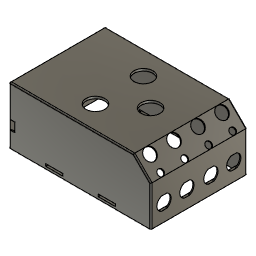
Main_case (Autodesk Fusion 360 design; units mm, degrees)
Autodesk Fusion 360 part; units mm, degrees
note: some values were not read from the file. Set by a fixed rule: which sketch regions a step uses.
sketch "Sketch1" plane through (0, 0, 0) normal (0, 0, 1) x (1, 0, 0)
  line L0 (0, 0) -> (120, 0)
  line L1 (120, 0) -> (120, 80)
  line L2 (120, 80) -> (0, 80)
  line L3 (0, 80) -> (0, 0)
  line L4 (-2, -2) -> (-2, 82)
  line L5 (-2, 82) -> (122, 82)
  line L6 (122, 82) -> (122, -2)
  line L7 (122, -2) -> (-2, -2)
  constraint horizontal L0
  constraint vertical L1
  constraint horizontal L2
  constraint vertical L3
  constraint coincident L0.start L3.end
  constraint perpendicular L4 L5
  constraint perpendicular L4 L7
extrude "Extrude1" add sketch "Sketch1" along normal blind 40 makes body 1
extrude "Extrude2" add 1 faces at (40, 81.3333, 40) along direction (0, 0, 1) blind 10 on bodies 1 bodies 1
sketch "Sketch2" plane through (0, -2, 0) normal (0, -1, 0) x (1, 0, 0)
  line L0 (-2, 0) -> (122, 0)
  line L1 (122, 0) -> (122, 50)
  line L2 (122, 50) -> (-2, 50)
  line L3 (-2, 50) -> (-2, 0)
  line L4 (122, 35) -> (107, 50)
  constraint coincident L2 L4.end
  constraint coincident L1 L4.start
extrude "Extrude3" cut sketch "Sketch2" against normal blind 135 contours L1 L2 L4 bodies 1
sketch "Sketch3" plane through (78.5, 0, 78.5) normal (0.707107, 0, 0.707107) x (0, 1, 0)
  line L0 (80, -40.3051) -> (80, -58.6899)
  line L1 (80, -58.6899) -> (0, -58.6899)
  line L2 (0, -58.6899) -> (0, -40.3051)
  line L3 (0, -40.3051) -> (-2, -40.3051)
  line L4 (-2, -40.3051) -> (-2, -61.5183)
  line L5 (-2, -61.5183) -> (82, -61.5183)
  line L6 (82, -61.5183) -> (82, -40.3051)
  line L7 (82, -40.3051) -> (80, -40.3051)
  line L8 (-2, -40.3051) -> (82, -40.3051)
  line L9 (82, -40.3051) -> (82, -61.5183)
  line L10 (82, -61.5183) -> (-2, -61.5183)
  line L11 (-2, -61.5183) -> (-2, -40.3051)
  constraint horizontal L8
  constraint vertical L9
  constraint horizontal L10
  constraint vertical L11
  constraint coincident L5.end L6.start
  constraint coincident L3.end L4.start
extrude "Extrude4" add sketch "Sketch3" against normal blind 2 bodies 1
sketch "Sketch4" plane through (0, 0, 50) normal (0, 0, 1) x (-1, 0, 0)
  line L0 (-107, -80) -> (-107, -82)
  line L1 (-107, -82) -> (2, -82)
  line L2 (2, -82) -> (2, 2)
  line L3 (2, 2) -> (-107, 2)
  line L4 (-107, 2) -> (-107, 0)
  line L5 (-107, 0) -> (0, 0)
  line L6 (0, 0) -> (0, -80)
  line L7 (0, -80) -> (-107, -80)
  line L8 (2, -82) -> (-107, -82)
  line L9 (-107, -82) -> (-107, 2)
  line L10 (-107, 2) -> (2, 2)
  line L11 (2, 2) -> (2, -82)
  constraint horizontal L8
  constraint vertical L9
  constraint horizontal L10
  constraint vertical L11
  constraint coincident L3.end L4.start
  constraint coincident L1.end L2.start
extrude "Extrude5" add sketch "Sketch4" against normal blind 2 bodies 1
sketch "Sketch5" plane through (78.5, 0, 78.5) normal (0.707107, 0, 0.707107) x (0, 1, 0)
  line L0 (82, -40.3051) -> (-2, -40.3051)
  line L1 (-2, -40.3051) -> (-2, -61.5183)
  line L2 (-2, -61.5183) -> (82, -61.5183)
  line L3 (82, -61.5183) -> (82, -40.3051)
  line L4 (-2, -40.3051) -> (-2, -61.5183)
  line L5 (-2, -40.3051) -> (-2, -50.9117)
  line L6 (40, -40.3051) -> (-2, -40.3051)
  line L7 (82, -40.3051) -> (40, -40.3051)
  line L8 (-2, -40.3051) -> (19, -40.3051)
  circle A0 centre (8.5, -58.7683) radius 2.75
  circle A1 centre (8.5, -45.5551) radius 5.25
  line L9 (19, -40.3051) -> (40, -40.3051)
  circle A2 centre (29.5, -45.5551) radius 5.25
  circle A3 centre (29.5, -58.7683) radius 2.75
  line L10 (40, -40.3051) -> (61, -40.3051)
  line L11 (61, -40.3051) -> (82, -40.3051)
  circle A4 centre (50.5, -45.5551) radius 5.25
  circle A5 centre (50.5, -58.7683) radius 2.75
  circle A6 centre (71.5, -45.5551) radius 5.25
  circle A7 centre (71.5, -58.7683) radius 2.75
  dimension "d13" = 5.5
  dimension "d14" = 10.5
  dimension "d15" = 10.5
  dimension "d16" = 5.5
  dimension "d17" = 10.5
  dimension "d18" = 5.5
  dimension "d19" = 10.5
  dimension "d20" = 5.5
  constraint coincident L0.end L1.start
  constraint coincident L1.end L2.start
  constraint midpoint L4 L5.end
  constraint midpoint L0 L6.start
  constraint midpoint L6 L8.end
  constraint coincident L0.start L3.end
  constraint midpoint L7 L10.end
  measures "d13" diameter of A0
  measures "d14" diameter of A1
  measures "d15" diameter of A2
  measures "d16" diameter of A3
  measures "d17" diameter of A4
  measures "d18" diameter of A5
  measures "d19" diameter of A6
  measures "d20" diameter of A7
extrude "Extrude6" cut sketch "Sketch5" against normal blind 20 contours A6 | A4 | A2 | A1 | A0 | A3 | A5 | A7 bodies 1
chamfer "Chamfer1" distance 1 angle 45 16 edges at (105, 71.5, 48) (113.0104, 71.5, 41.1612) (116.6967, 71.5, 37.4749) (120, 71.5, 33) (105, 50.5, 48) (113.0104, 50.5, 41.1612) (116.6967, 50.5, 37.4749) (120, 50.5, 33) (105, 29.5, 48) (113.0104, 29.5, 41.1612) (116.6967, 29.5, 37.4749) (120, 29.5, 33) (105, 8.5, 48) (113.0104, 8.5, 41.1612) (116.6967, 8.5, 37.4749) (120, 8.5, 33) on bodies 1
sketch "Sketch6" plane through (120, 0, 0) normal (-1, 0, 0) x (0, -1, 0)
  spline S0 degree 3 poles (-11.6272, 34.1716) (-11.364, 33.6522) (-11.0186, 33.1887) (-10.2377, 32.5093) (-9.8211, 32.2678) (-9.0887, 32.0448) (-8.7945, 32) (-8.5, 32) (-8.2055, 32) (-7.9113, 32.0448) (-7.1789, 32.2678) (-6.7623, 32.5093) (-5.9814, 33.1887) (-5.636, 33.6522) (-5.3728, 34.1716) knots -0.948969 -0.948969 -0.948969 -0.948969 -0.551543 -0.551543 -0.212132 -0.212132 0 0 0 0.212132 0.212132 0.551543 0.551543 0.948969 0.948969 0.948969 0.948969
  spline S1 degree 3 poles (-11.6784, 34.2753) (-11.6617, 34.2405) (-11.6446, 34.2059) (-11.6272, 34.1716) knots -0.975231 -0.975231 -0.975231 -0.975231 -0.948969 -0.948969 -0.948969 -0.948969
  spline S2 degree 2 poles (-11.7203, 34.1716) (-11.6993, 34.2238) (-11.6784, 34.2753) knots -18.7019 -18.7019 -18.7019 -18.668651 -18.668651 -18.668651 weights 1.000003 1.000003 1.000003
  line L0 (-11.7203, 34.1716) -> (-26.2797, 34.1716)
  spline S3 degree 2 poles (-26.3216, 34.2753) (-26.3007, 34.2238) (-26.2797, 34.1716) knots -13.625289 -13.625289 -13.625289 -13.59204 -13.59204 -13.59204 weights 1.000003 1.000003 1.000003
  spline S4 degree 3 poles (-26.3216, 34.2753) (-26.3383, 34.2405) (-26.3554, 34.2059) (-26.3728, 34.1716) knots -0.975231 -0.975231 -0.975231 -0.975231 -0.948969 -0.948969 -0.948969 -0.948969
  spline S5 degree 3 poles (-32.6272, 34.1716) (-32.364, 33.6522) (-32.0186, 33.1887) (-31.2377, 32.5093) (-30.8211, 32.2678) (-30.0887, 32.0448) (-29.7945, 32) (-29.5, 32) (-29.2055, 32) (-28.9113, 32.0448) (-28.1789, 32.2678) (-27.7623, 32.5093) (-26.9814, 33.1887) (-26.636, 33.6522) (-26.3728, 34.1716) knots -0.948969 -0.948969 -0.948969 -0.948969 -0.551543 -0.551543 -0.212132 -0.212132 0 0 0 0.212132 0.212132 0.551543 0.551543 0.948969 0.948969 0.948969 0.948969
  spline S6 degree 3 poles (-32.6784, 34.2753) (-32.6617, 34.2405) (-32.6446, 34.2059) (-32.6272, 34.1716) knots -0.975231 -0.975231 -0.975231 -0.975231 -0.948969 -0.948969 -0.948969 -0.948969
  spline S7 degree 2 poles (-32.7203, 34.1716) (-32.6993, 34.2238) (-32.6784, 34.2753) knots -18.7019 -18.7019 -18.7019 -18.668651 -18.668651 -18.668651 weights 1.000003 1.000003 1.000003
  line L1 (-32.7203, 34.1716) -> (-47.2797, 34.1716)
  spline S8 degree 2 poles (-47.3216, 34.2753) (-47.3007, 34.2238) (-47.2797, 34.1716) knots -13.625289 -13.625289 -13.625289 -13.59204 -13.59204 -13.59204 weights 1.000003 1.000003 1.000003
  spline S9 degree 3 poles (-47.3216, 34.2753) (-47.3383, 34.2405) (-47.3554, 34.2059) (-47.3728, 34.1716) knots -0.975231 -0.975231 -0.975231 -0.975231 -0.948969 -0.948969 -0.948969 -0.948969
  spline S10 degree 3 poles (-53.6272, 34.1716) (-53.364, 33.6522) (-53.0186, 33.1887) (-52.2377, 32.5093) (-51.8211, 32.2678) (-51.0887, 32.0448) (-50.7945, 32) (-50.5, 32) (-50.2055, 32) (-49.9113, 32.0448) (-49.1789, 32.2678) (-48.7623, 32.5093) (-47.9814, 33.1887) (-47.636, 33.6522) (-47.3728, 34.1716) knots -0.948969 -0.948969 -0.948969 -0.948969 -0.551543 -0.551543 -0.212132 -0.212132 0 0 0 0.212132 0.212132 0.551543 0.551543 0.948969 0.948969 0.948969 0.948969
  spline S11 degree 3 poles (-53.6784, 34.2753) (-53.6617, 34.2405) (-53.6446, 34.2059) (-53.6272, 34.1716) knots -0.975231 -0.975231 -0.975231 -0.975231 -0.948969 -0.948969 -0.948969 -0.948969
  spline S12 degree 2 poles (-53.7203, 34.1716) (-53.6993, 34.2238) (-53.6784, 34.2753) knots -18.7019 -18.7019 -18.7019 -18.668651 -18.668651 -18.668651 weights 1.000003 1.000003 1.000003
  line L2 (-53.7203, 34.1716) -> (-68.2797, 34.1716)
  spline S13 degree 2 poles (-68.3216, 34.2753) (-68.3007, 34.2238) (-68.2797, 34.1716) knots -13.625289 -13.625289 -13.625289 -13.59204 -13.59204 -13.59204 weights 1.000003 1.000003 1.000003
  spline S14 degree 3 poles (-68.3216, 34.2753) (-68.3383, 34.2405) (-68.3554, 34.2059) (-68.3728, 34.1716) knots -0.975231 -0.975231 -0.975231 -0.975231 -0.948969 -0.948969 -0.948969 -0.948969
  spline S15 degree 3 poles (-74.6272, 34.1716) (-74.364, 33.6522) (-74.0186, 33.1887) (-73.2377, 32.5093) (-72.8211, 32.2678) (-72.0887, 32.0448) (-71.7945, 32) (-71.5, 32) (-71.2055, 32) (-70.9113, 32.0448) (-70.1789, 32.2678) (-69.7623, 32.5093) (-68.9814, 33.1887) (-68.636, 33.6522) (-68.3728, 34.1716) knots -0.948969 -0.948969 -0.948969 -0.948969 -0.551543 -0.551543 -0.212132 -0.212132 0 0 0 0.212132 0.212132 0.551543 0.551543 0.948969 0.948969 0.948969 0.948969
  spline S16 degree 3 poles (-74.6784, 34.2753) (-74.6617, 34.2405) (-74.6446, 34.2059) (-74.6272, 34.1716) knots -0.975231 -0.975231 -0.975231 -0.975231 -0.948969 -0.948969 -0.948969 -0.948969
  spline S17 degree 2 poles (-74.7203, 34.1716) (-74.6993, 34.2238) (-74.6784, 34.2753) knots -18.7019 -18.7019 -18.7019 -18.668651 -18.668651 -18.668651 weights 1.000003 1.000003 1.000003
  line L3 (-74.7203, 34.1716) -> (-80, 34.1716)
  line L4 (-80, 34.1716) -> (-80, 0)
  line L5 (-80, 0) -> (0, 0)
  line L6 (0, 0) -> (0, 34.1716)
  line L7 (0, 34.1716) -> (-5.2797, 34.1716)
  spline S18 degree 2 poles (-5.3216, 34.2753) (-5.3007, 34.2238) (-5.2797, 34.1716) knots -13.625289 -13.625289 -13.625289 -13.59204 -13.59204 -13.59204 weights 1.000003 1.000003 1.000003
  spline S19 degree 3 poles (-5.3216, 34.2753) (-5.3383, 34.2405) (-5.3554, 34.2059) (-5.3728, 34.1716) knots -0.975231 -0.975231 -0.975231 -0.975231 -0.948969 -0.948969 -0.948969 -0.948969
  circle A0 centre (-70.5, 15) radius 6.25
  circle A1 centre (-50.5, 15) radius 6.25
  circle A2 centre (-29.5, 15) radius 6.25
  circle A3 centre (-9.5, 15) radius 6.25
  line L8 (-63.25, 9.25) -> (-77.75, 9.25)
  line L9 (-77.75, 9.25) -> (-77.75, 20.75)
  line L10 (-77.75, 20.75) -> (-63.25, 20.75)
  line L11 (-63.25, 20.75) -> (-63.25, 9.25)
  line L12 (-43.25, 9.25) -> (-57.75, 9.25)
  line L13 (-57.75, 9.25) -> (-57.75, 20.75)
  line L14 (-57.75, 20.75) -> (-43.25, 20.75)
  line L15 (-43.25, 20.75) -> (-43.25, 9.25)
  line L16 (-22.25, 9.25) -> (-36.75, 9.25)
  line L17 (-36.75, 9.25) -> (-36.75, 20.75)
  line L18 (-36.75, 20.75) -> (-22.25, 20.75)
  line L19 (-22.25, 20.75) -> (-22.25, 9.25)
  line L20 (-2.25, 9.25) -> (-16.75, 9.25)
  line L21 (-16.75, 9.25) -> (-16.75, 20.75)
  line L22 (-16.75, 20.75) -> (-2.25, 20.75)
  line L23 (-2.25, 20.75) -> (-2.25, 9.25)
  point P0 (-70.5, 15)
  point P1 (-50.5, 15)
  point P2 (-29.5, 15)
  point P3 (-9.5, 15)
  constraint horizontal L8
  constraint perpendicular L8 L9
  constraint parallel L8 L10
  constraint parallel L9 L11
  constraint horizontal L12
  constraint perpendicular L12 L13
  constraint parallel L12 L14
  constraint parallel L13 L15
  constraint coincident P1 A1.centre
  constraint horizontal L16
  constraint perpendicular L16 L17
  constraint parallel L16 L18
  constraint parallel L17 L19
  constraint coincident P2 A2.centre
  constraint horizontal L20
  constraint perpendicular L20 L21
  constraint parallel L20 L22
  constraint parallel L21 L23
  constraint coincident P3 A3.centre
extrude "Extrude7" cut sketch "Sketch6" against normal blind 51 contours A0 L8 L10 | A1 L12 L14 | A2 L16 L18 | A3 L20 L22 bodies 1
extrude "Extrude8" cut sketch "Sketch6" against normal blind 1 contours A0 L8 L10 L11 | A0 L8 L9 L10 | A1 L12 L14 L15 | A1 L12 L13 L14 | A2 L16 L18 L19 | A2 L16 L17 L18 | A3 L20 L22 L23 | A3 L20 L21 L22 bodies 1
sketch "Sketch7" plane through (0, 0, 50) normal (0, 0, 1) x (-1, 0, 0)
  line L0 (-107, 2) -> (-107, -8.5)
  line L1 (-107, -8.5) -> (-107, -29.5)
  line L2 (-107, -29.5) -> (-107, -50.5)
  line L3 (-107, -50.5) -> (-107, -71.5)
  line L4 (-107, -71.5) -> (-107, -82)
  line L5 (-107, -82) -> (2, -82)
  line L6 (2, -82) -> (2, 2)
  line L7 (2, 2) -> (-107, 2)
  line L8 (-107, -82) -> (-107, 2)
  line L9 (-107, -40) -> (2, -40)
  line L10 (-52.5, -40) -> (-52.5, 2)
  line L11 (-52.5, -40) -> (-52.5, -82)
  circle A0 centre (-52.5, -61) radius 8.25
  circle A1 centre (-52.5, -19) radius 8.25
  line L12 (-107, -40) -> (-52.5, -40)
  circle A2 centre (-79.75, -40) radius 8.25
  dimension "d42" = 16.5
  dimension "d43" = 16.5
  dimension "d75" = 16.5
  constraint coincident L4.end L5.start
  constraint coincident L0.start L7.end
  constraint midpoint L8 L9.start
  constraint midpoint L6 L9.end
  constraint midpoint L9 L10.start
  constraint midpoint L7 L10.end
  constraint midpoint L5 L11.end
  constraint midpoint L11 A0.centre
  constraint midpoint L10 A1.centre
  constraint midpoint L12 A2.centre
  measures "d42" diameter of A0
  measures "d43" diameter of A1
  measures "d75" diameter of A2
extrude "Extrude9" cut sketch "Sketch7" against normal blind 30 contours L10 A1 | L10 A1 | L11 A0 | L11 A0 bodies 1
sketch "Sketch8" plane through (0, 0, 0) normal (1, 0, 0) x (0, 1, 0)
  line L0 (80, 48) -> (0, 48)
  line L1 (0, 48) -> (0, 0)
  line L2 (0, 0) -> (80, 0)
  line L3 (80, 0) -> (80, 48)
  line L4 (10, 26.75) -> (0, 26.75)
  line L5 (10, 9.25) -> (0, 9.25)
  line L6 (0, 26.75) -> (27.5, 26.75)
  line L7 (0, 9.25) -> (27.5, 9.25)
  line L8 (27.5, 26.75) -> (27.5, 9.25)
  line L9 (27.5, 26.75) -> (22.4893, 26.75)
  line L10 (22.4893, 26.75) -> (22.4893, 9.25)
  line L11 (22.4893, 9.25) -> (27.5, 9.25)
  line L12 (27.5, 9.25) -> (27.5, 26.75)
  line L13 (27.5, 18) -> (0, 18)
  line L14 (27.5, 18) -> (80, 18)
  line L15 (80, 18) -> (80, 27.75)
  line L16 (80, 18) -> (80, 8.25)
  line L17 (80, 18) -> (80, 23.5)
  line L18 (80, 18) -> (80, 12.5)
  dimension "d48" = 27.5
  dimension "d49" = 27.5
  dimension "d60" = 9.75
  dimension "d61" = 9.75
  dimension "d62" = 5.5
  dimension "d63" = 5.5
  constraint coincident L1 L4.end
  constraint perpendicular L1 L4
  constraint coincident L1 L5.end
  constraint perpendicular L1 L5
  constraint perpendicular L1 L6
  constraint perpendicular L1 L7
  constraint horizontal L9
  constraint vertical L10
  constraint horizontal L11
  constraint vertical L12
  constraint coincident L7 L10.end
  constraint midpoint L12 L13.start
  constraint coincident L1 L13.end
  constraint perpendicular L1 L13
  constraint coincident L3 L14.end
  constraint perpendicular L3 L14
  constraint perpendicular L14 L15
  constraint perpendicular L14 L16
  constraint perpendicular L14 L17
  constraint perpendicular L14 L18
  measures "d48" distance of L4.end L6.end
  measures "d49" distance of L5.end L7.end
  measures "d60" distance of L14.end L15.end
  measures "d61" distance of L14.end L16.end
  measures "d62" distance of L14.end L17.end
  measures "d63" distance of L14.end L18.end
extrude "Extrude10" cut sketch "Sketch8" against normal blind 1.2 contours L7 L8 L10 L11 L12 L13 | L6 L8 L9 L10 L12 L13 bodies 1
extrude "Extrude11" cut sketch "Sketch8" against normal blind 1 contours L1 L4 L6 L10 L13 | L1 L5 L7 L10 L13 bodies 1
sketch "Sketch9" plane through (0, 0, 0) normal (0, 1, 0) x (-1, 0, 0)
  line L0 (0, 48) -> (-106.1716, 48)
  line L1 (-106.1716, 48) -> (-120, 34.1716)
  line L2 (-120, 34.1716) -> (-120, 0)
  line L3 (-120, 0) -> (0, 0)
  line L4 (0, 0) -> (0, 9.25)
  line L5 (0, 9.25) -> (1, 9.25)
  line L6 (1, 9.25) -> (1, 26.75)
  line L7 (1, 26.75) -> (0, 26.75)
  line L8 (0, 26.75) -> (0, 48)
  line L9 (1, 26.75) -> (-3, 26.75)
  line L10 (-3, 26.75) -> (-3, 9.25)
  line L11 (-3, 9.25) -> (1, 9.25)
  line L12 (1, 9.25) -> (1, 26.75)
  line L13 (1, 18) -> (1, 22)
  line L14 (1, 18) -> (1, 14)
  line L15 (1, 22) -> (-3, 22)
  line L16 (1, 14) -> (-3, 14)
  dimension "d54" = 4
  dimension "d55" = 17.5
  constraint horizontal L9
  constraint vertical L10
  constraint horizontal L11
  constraint vertical L12
  constraint coincident L6.end L7.start
  constraint midpoint L12 L13.start
  constraint coincident L6 L13.end
  constraint parallel L6 L13
  constraint coincident L12 L14.end
  constraint parallel L12 L14
  constraint coincident L10 L15.end
  constraint perpendicular L10 L15
  constraint coincident L10 L16.end
  constraint perpendicular L10 L16
  measures "d54" distance of L6.end L9.end
  measures "d55" distance of L6.end L5.end
extrude "Extrude12" cut sketch "Sketch9" against normal blind 1 contours L6 L7 L9 L10 L12 L15 | L5 L6 L10 L11 L12 L16 bodies 1
extrude "Extrude13" cut sketch "Sketch9" against normal blind 9 contours L6 L10 L12 L13 L14 L15 L16 bodies 1
sketch "Sketch10" plane through (0, 80, 0) normal (0, -1, 0) x (1, 0, 0)
  line L0 (106.1716, 48) -> (0, 48)
  line L1 (0, 48) -> (0, 0)
  line L2 (0, 0) -> (120, 0)
  line L3 (120, 0) -> (120, 34.1716)
  line L4 (120, 34.1716) -> (106.1716, 48)
  line L5 (0, 8.25) -> (3.5, 8.25)
  line L6 (0, 27.75) -> (3.5, 27.75)
  line L7 (0, 23.5) -> (3.5, 23.5)
  line L8 (0, 12.5) -> (3.5, 12.5)
  line L9 (3.5, 27.75) -> (3.5, 8.25)
  dimension "d67" = 3.5
  dimension "d68" = 3.5
  constraint coincident L1 L5.start
  constraint perpendicular L1 L5
  constraint coincident L1 L6.start
  constraint perpendicular L1 L6
  constraint coincident L1 L7.start
  constraint perpendicular L1 L7
  constraint coincident L1 L8.start
  constraint perpendicular L1 L8
  constraint perpendicular L5 L9
  measures "d67" distance of L7.start L7.end
  measures "d68" distance of L8.start L8.end
extrude "Extrude14" cut sketch "Sketch10" against normal blind 1 contours L1 L6 L7 L9 | L1 L5 L8 L9 bodies 1
extrude "Extrude15" cut sketch "Sketch10" against normal blind 10 contours L1 L7 L8 L9 bodies 1
sketch "Sketch11" plane through (0, 0, 0) normal (1, 0, 0) x (0, 1, 0)
  line L0 (27.5, 9.25) -> (0, 9.25)
  line L1 (0, 9.25) -> (0, 0)
  line L2 (0, 0) -> (80, 0)
  line L3 (80, 0) -> (80, 8.25)
  line L4 (80, 8.25) -> (81, 8.25)
  line L5 (81, 8.25) -> (81, 12.5)
  line L6 (81, 12.5) -> (82, 12.5)
  line L7 (82, 12.5) -> (82, 23.5)
  line L8 (82, 23.5) -> (81, 23.5)
  line L9 (81, 23.5) -> (81, 27.75)
  line L10 (81, 27.75) -> (80, 27.75)
  line L11 (80, 27.75) -> (80, 48)
  line L12 (80, 48) -> (0, 48)
  line L13 (0, 48) -> (0, 26.75)
  line L14 (0, 26.75) -> (27.5, 26.75)
  line L15 (27.5, 26.75) -> (27.5, 9.25)
  line L16 (81, 23.5) -> (76, 23.5)
  line L17 (76, 23.5) -> (76, 12.5)
  line L18 (76, 12.5) -> (81, 12.5)
  line L19 (81, 27.75) -> (80.5, 27.75)
  line L20 (80.5, 27.75) -> (80.5, 8.25)
  line L21 (81, 23.5) -> (81, 12.5)
  constraint coincident L8.end L9.start
  constraint perpendicular L9 L16
  constraint perpendicular L6 L17
  constraint coincident L5.end L6.start
  constraint perpendicular L5 L18
  constraint coincident L9.end L10.start
  constraint midpoint L10 L19.end
  constraint midpoint L4 L20.end
extrude "Extrude16" cut sketch "Sketch11" against normal blind 1 contours L4 L5 L18 L20 | L16 L18 L20 L21 | L16 L17 L18 L20 | L9 L10 L16 L19 L20 bodies 1
extrude "Extrude17" cut sketch "Sketch7" against normal blind 5 contours L9 L12 A2 | L9 L12 A2 bodies 1
extrude "Extrude18" add sketch "Sketch1" against normal blind 2 separate body contours L0 L1 L2 L3 | L4 L5 L6 L7 makes body 2
sketch "Sketch12" plane through (0, 0, 0) normal (0, 0, 1) x (1, 0, 0)
  line L0 (2, 78) -> (118, 78)
  line L1 (118, 78) -> (118, 2)
  line L2 (118, 2) -> (2, 2)
  line L3 (2, 2) -> (2, 78)
  line L4 (2, 78) -> (118, 78)
  line L5 (118, 78) -> (118, 2)
  line L6 (118, 2) -> (2, 2)
  line L7 (2, 2) -> (2, 78)
  constraint perpendicular L0 L1
  constraint perpendicular L1 L2
  constraint perpendicular L0 L3
  constraint horizontal L4
  constraint vertical L5
  constraint horizontal L6
  constraint vertical L7
extrude "Extrude19" add sketch "Sketch1" along normal blind 2 contours L0 L1 L2 L3 bodies 2
sketch "Sketch13" plane through (0, 0, 2) normal (0, 0, 1) x (-1, 0, 0)
  line L0 (0, -80) -> (0, 0)
  line L1 (0, 0) -> (-120, 0)
  line L2 (-120, 0) -> (-120, -80)
  line L3 (-120, -80) -> (0, -80)
  line L4 (-2, -78) -> (-118, -78)
  line L5 (-118, -78) -> (-118, -2)
  line L6 (-118, -2) -> (-2, -2)
  line L7 (-2, -2) -> (-2, -78)
  constraint horizontal L4
  constraint vertical L5
  constraint horizontal L6
  constraint vertical L7
extrude "Extrude20" cut sketch "Sketch13" against normal blind 2 contours L4 L5 L6 L7 bodies 2
fillet "Fillet1" radius 1 9 edges at (-2, 82, 25) (52.5, 82, 50) (-2, 40, 50) (52.5, -2, 50) (114.5, -2, 42.5) (114.5, 82, 42.5) (122, 82, 17.5) (122, -2, 17.5) (-2, -2, 25) on bodies 1
fillet "Fillet2" radius 1 8 edges at (-2, 82, -1) (-2, 40, -2) (60, 82, -2) (-2, -2, -1) (60, -2, -2) (122, -2, -1) (122, 40, -2) (122, 82, -1) on bodies 2
sketch "Sketch14" plane through (0, 0, 2) normal (0, 0, 1) x (-1, 0, 0)
  line L0 (-118, -78) -> (-118, -2)
  line L1 (-118, -2) -> (-2, -2)
  line L2 (-2, -2) -> (-2, -78)
  line L3 (-2, -78) -> (-118, -78)
  line L4 (0, -80) -> (0, 0)
  line L5 (0, 0) -> (-120, 0)
  line L6 (-120, 0) -> (-120, -80)
  line L7 (-120, -80) -> (0, -80)
  line L8 (-118, -40) -> (-118, -55)
  line L9 (-118, -40) -> (-118, -25)
  line L10 (-118, -25) -> (-120, -25)
  line L11 (-120, -25) -> (-120, -55)
  line L12 (-118, -55) -> (-120, -55)
  line L13 (-30, -2) -> (-45, -2)
  line L14 (-45, -2) -> (-45, 0)
  line L15 (-45, 0) -> (-30, 0)
  line L16 (-30, 0) -> (-30, -2)
  line L17 (-76, -2) -> (-91, -2)
  line L18 (-91, -2) -> (-91, 0)
  line L19 (-91, 0) -> (-76, 0)
  line L20 (-76, 0) -> (-76, -2)
  line L21 (-2, -40) -> (-2, -47.5)
  line L22 (-2, -47.5) -> (0, -47.5)
  line L23 (0, -47.5) -> (0, -32.5)
  line L24 (-2, -32.5) -> (0, -32.5)
  line L25 (-2, -32.5) -> (-2, -40)
  line L26 (-30, -80) -> (-45, -80)
  line L27 (-45, -80) -> (-45, -78)
  line L28 (-45, -78) -> (-30, -78)
  line L29 (-30, -78) -> (-30, -80)
  line L30 (-76, -80) -> (-91, -80)
  line L31 (-91, -80) -> (-91, -78)
  line L32 (-91, -78) -> (-76, -78)
  line L33 (-76, -78) -> (-76, -80)
  constraint midpoint L0 L8.start
  constraint coincident L0 L8.end
  constraint parallel L0 L8
  constraint coincident L0 L9.end
  constraint parallel L0 L9
  constraint coincident L6 L10.end
  constraint perpendicular L6 L10
  constraint coincident L6 L11.end
  constraint perpendicular L10 L11
  constraint perpendicular L11 L12
  constraint horizontal L13
  constraint vertical L14
  constraint horizontal L15
  constraint vertical L16
  constraint coincident L5 L14.end
  constraint coincident L1 L13.start
  constraint horizontal L17
  constraint vertical L18
  constraint horizontal L19
  constraint vertical L20
  constraint coincident L5 L18.end
  constraint coincident L1 L17.start
  constraint midpoint L2 L21.start
  constraint coincident L2 L21.end
  constraint parallel L2 L21
  constraint coincident L4 L22.end
  constraint perpendicular L4 L22
  constraint coincident L4 L23.end
  constraint perpendicular L22 L23
  constraint coincident L2 L24.start
  constraint perpendicular L23 L24
  constraint coincident L7 L26.start
  constraint coincident L7 L30.start
  constraint horizontal L26
  constraint vertical L27
  constraint horizontal L28
  constraint vertical L29
  constraint coincident L3 L27.end
  constraint horizontal L30
  constraint vertical L31
  constraint horizontal L32
  constraint vertical L33
  constraint coincident L3 L31.end
extrude "Extrude21" add sketch "Sketch14" along normal blind 2 contours L0 L6 L8 L9 L10 L11 L12 | L3 L7 L30 L31 L32 L33 | L3 L7 L26 L27 L28 L29 | L1 L5 L17 L18 L19 L20 | L2 L4 L21 L22 L23 L24 L25 | L1 L5 L13 L14 L15 L16 bodies 2
sketch "Sketch15" plane through (120, 0, 0) normal (1, 0, 0) x (0, 1, 0)
  line L0 (0, 0) -> (80, 0)
  line L1 (80, 0) -> (80, 2)
  line L2 (80, 2) -> (55, 2)
  line L3 (55, 2) -> (55, 4)
  line L4 (55, 4) -> (25, 4)
  line L5 (25, 4) -> (25, 2)
  line L6 (25, 2) -> (0, 2)
  line L7 (0, 2) -> (0, 0)
  line L8 (25, 2) -> (55, 2)
  constraint coincident L5.end L6.start
  constraint coincident L2.end L3.start
extrude "Extrude22" add sketch "Sketch15" along normal blind 1 contours L3 L4 L5 L8 bodies 2
sketch "Sketch16" plane through (0, 0, 0) normal (0, -1, 0) x (1, 0, 0)
  line L0 (0, 0) -> (120, 0)
  line L1 (120, 0) -> (120, 2)
  line L2 (120, 2) -> (91, 2)
  line L3 (91, 2) -> (91, 4)
  line L4 (91, 4) -> (76, 4)
  line L5 (76, 4) -> (76, 2)
  line L6 (76, 2) -> (45, 2)
  line L7 (45, 2) -> (45, 4)
  line L8 (45, 4) -> (30, 4)
  line L9 (30, 4) -> (30, 2)
  line L10 (30, 2) -> (0, 2)
  line L11 (0, 2) -> (0, 0)
  line L12 (30, 2) -> (91, 2)
  constraint coincident L9.end L10.start
  constraint coincident L2.end L3.start
extrude "Extrude23" add sketch "Sketch16" along normal blind 2 contours L7 L8 L9 L12 | L3 L4 L5 L12 bodies 2
sketch "Sketch17" plane through (0, 0, 0) normal (-1, 0, 0) x (0, -1, 0)
  line L0 (-80, 0) -> (0, 0)
  line L1 (0, 0) -> (0, 2)
  line L2 (0, 2) -> (-32.5, 2)
  line L3 (-32.5, 2) -> (-32.5, 4)
  line L4 (-32.5, 4) -> (-47.5, 4)
  line L5 (-47.5, 4) -> (-47.5, 2)
  line L6 (-47.5, 2) -> (-80, 2)
  line L7 (-80, 2) -> (-80, 0)
  line L8 (-55.0095, 2) -> (-32.5, 2)
  constraint coincident L6 L8.start
  constraint coincident L2.end L3.start
  constraint perpendicular L3 L8
extrude "Extrude24" add sketch "Sketch17" along normal blind 2 contours L3 L4 L5 L8 bodies 2
sketch "Sketch18" plane through (0, 80, 0) normal (0, 1, 0) x (-1, 0, 0)
  line L0 (-120, 0) -> (0, 0)
  line L1 (0, 0) -> (0, 2)
  line L2 (0, 2) -> (-30, 2)
  line L3 (-30, 2) -> (-30, 4)
  line L4 (-30, 4) -> (-45, 4)
  line L5 (-45, 4) -> (-45, 2)
  line L6 (-45, 2) -> (-76, 2)
  line L7 (-76, 2) -> (-76, 4)
  line L8 (-76, 4) -> (-91, 4)
  line L9 (-91, 4) -> (-91, 2)
  line L10 (-91, 2) -> (-120, 2)
  line L11 (-120, 2) -> (-120, 0)
  line L12 (-91, 2) -> (-30, 2)
  constraint coincident L9.end L10.start
  constraint coincident L2.end L3.start
extrude "Extrude25" add sketch "Sketch18" along normal blind 2 contours L7 L8 L9 L12 | L3 L4 L5 L12 bodies 2
copy_body "CopyPasteBodies1" bodies 2 makes body 3
move_body "Move1" bodies 3 to x (1, 0, 0) y (0, 1, 0) z (0, 0, 1) at (0, 0, 0)
combine "Combine1" operation cut target body 1 tool bodies 3
extrude "Extrude26" cut 1 faces at (120, 45, 4) along direction (0, 0, -1) blind 0.5 on bodies 2 bodies 2
extrude "Extrude27" cut 1 faces at (119.6667, 25, 3) along direction (0, 1, 0) blind 0.5 on bodies 2 bodies 2
extrude "Extrude28" cut 1 faces at (119.6667, 55, 3) along direction (0, -1, 0) blind 0.5 on bodies 2 bodies 2
sketch "Sketch19" plane through (91, 0, 0) normal (1, 0, 0) x (0, 1, 0)
  line L0 (0, 2) -> (2, 2)
  line L1 (2, 2) -> (2, 4)
  line L2 (2, 4) -> (-2, 4)
  line L3 (-2, 4) -> (-2, 2)
  line L4 (-2, 2) -> (0, 2)
  line L5 (0, 4) -> (-1, 2)
  constraint midpoint L2 L5.start
  constraint midpoint L4 L5.end
extrude "Extrude29" cut sketch "Sketch19" against normal blind 270.3 contours L2 L3 L4 L5 bodies 2
extrude "Extrude30" cut 1 faces at (76, 0.6667, 2.6667) along direction (1, 0, 0) blind 0.5 on bodies 2 bodies 2
extrude "Extrude31" cut 1 faces at (30, 0.6667, 2.6667) along direction (1, 0, 0) blind 0.5 on bodies 2 bodies 2
extrude "Extrude32" cut 1 faces at (45, 0.6667, 2.6667) along direction (-1, 0, 0) blind 0.5 on bodies 2 bodies 2
extrude "Extrude33" cut 1 faces at (91, 0.6667, 2.6667) along direction (-1, 0, 0) blind 0.5 on bodies 2 bodies 2
sketch "Sketch20" plane through (30, 0, 0) normal (-1, 0, 0) x (0, -1, 0)
  line L0 (-80, 2) -> (-78, 2)
  line L1 (-78, 2) -> (-78, 4)
  line L2 (-78, 4) -> (-82, 4)
  line L3 (-82, 4) -> (-82, 2)
  line L4 (-82, 2) -> (-80, 2)
  line L5 (-80, 4) -> (-81, 2)
  constraint midpoint L2 L5.start
  constraint midpoint L4 L5.end
extrude "Extrude34" cut sketch "Sketch20" against normal blind 408.5 contours L2 L3 L4 L5 bodies 2
extrude "Extrude35" cut 1 faces at (30, 79.3333, 3.3333) along direction (1, 0, 0) blind 0.5 on bodies 2 bodies 2
extrude "Extrude36" cut 1 faces at (76, 79.3333, 3.3333) along direction (1, 0, 0) blind 0.5 on bodies 2 bodies 2
extrude "Extrude37" cut 1 faces at (45, 79.3333, 3.3333) along direction (-1, 0, 0) blind 0.5 on bodies 2 bodies 2
extrude "Extrude38" cut 1 faces at (91, 79.3333, 3.3333) along direction (-1, 0, 0) blind 0.5 on bodies 2 bodies 2
sketch "Sketch21" plane through (0, 47.5, 0) normal (0, 1, 0) x (-1, 0, 0)
  line L0 (-2, 2) -> (0, 2)
  line L1 (0, 2) -> (2, 2)
  line L2 (2, 2) -> (2, 4)
  line L3 (2, 4) -> (-2, 4)
  line L4 (-2, 4) -> (-2, 2)
  line L5 (0, 4) -> (1, 2)
  constraint midpoint L3 L5.start
  constraint midpoint L1 L5.end
extrude "Extrude39" cut sketch "Sketch21" against normal blind 100 contours L1 L2 L3 L5 bodies 2
extrude "Extrude40" cut 1 faces at (0.6667, 32.5, 2.6667) along direction (0, 1, 0) blind 0.5 on bodies 2 bodies 2
extrude "Extrude41" cut 1 faces at (0.6667, 47.5, 2.6667) along direction (0, -1, 0) blind 0.5 on bodies 2 bodies 2
hidden bodies 2
